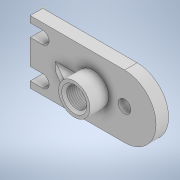
# Autodesk Inventor part: Деталь1
Saved by Autodesk Inventor 2020 (Build 240168000, 168)
## iProperties
Created: 2020-03-27
Part Number: Деталь1
Material: Типовые
Document SubType Name: Modeling
Designer: Trickster2038
Density: 1 g/cm^3
Appearance: По умолчанию
Mass: 46.5985 g
Surface Area: 144.743 cm^2
Volume: 46.5985 cm^3
Author: Trickster2038
Autodesk Inventor part; units mm, degrees
ref_plane "YZ Plane" through (0, 0, 0) normal (1, 0, 0) x (0, 1, 0)
sketch "Эскиз1" plane through (0, 0, 0) normal (0, 0, 1) x (1, 0, 0)
  line L0 (0, 0) -> (75, 0)
  line L1 (75, -50) -> (0, -50)
  line L2 (0, -50) -> (0, -45)
  arc A0 (75, -50) -> (75, 0) centre (75, -25) ccw
  line L3 (0, -25) -> (0, -15)
  line L4 (0, -15) -> (0, -35)
  line L5 (0, -35) -> (10, -35)
  line L6 (10, -45) -> (0, -45)
  line L7 (0, -15) -> (10, -15)
  line L8 (10, -5) -> (0, -5)
  arc A1 (10, -15) -> (10, -5) centre (10, -10) ccw
  arc A2 (10, -45) -> (10, -35) centre (10, -40) ccw
  line L9 (0, -5) -> (0, 0)
  line L10 (0, -35) -> (0, -15)
  circle A3 centre (50, -25) radius 12.5
  circle A4 centre (75, -25) radius 5
  line L11 (20, -25) -> (20, -21.5)
  line L12 (20, -21.5) -> (20, -28.5)
  line L13 (20, -28.5) -> (38, -28.5)
  line L14 (20, -21.5) -> (38, -21.5)
  constraints: 30 end point, 8 point on circle, 7 perpendicular, 5 centre point, 2 horizontal, 2 parallel, 1 coincident, 1 point on line, 1 vertical
sketch "Эскиз2" plane through (0, 0, 0) normal (0, 1, 0) x (-1, 0, 0)
  point P0 (0, 0)
sketch "Эскиз3" plane through (0, 0, 0) normal (0, 1, 0) x (-1, 0, 0)
  line L0 (0, 0) -> (0, 10)
  line L1 (0, 10) -> (-20, 10)
  line L2 (-20, 10) -> (-37.5, 10)
  line L3 (-37.5, 10) -> (-37.5, 20)
  line L4 (-37.5, 20) -> (-20, 10)
  line L5 (-44.031, 23.732) -> (-37.5, 20)
  line L6 (-44.031, 23.732) -> (-44.031, 33.732)
  line L7 (-44.031, 33.732) -> (-20, 33.732)
  line L8 (-20, 33.732) -> (-20, 10)
  dimension "d24" = 10
  dimension "d25" = 20
  dimension "d26" = 17.5
  dimension "d27" = 10
  dimension "d28" = 10
  constraints: 18 end point, 3 perpendicular, 2 point on line, 2 vertical, 1 collinear, 1 parallel
  measures "d24" distance of L0.start L0.end
  measures "d25" distance of L0.end L1.end
  measures "d26" distance of L1.end L2.end
  measures "d27" distance of L2.end L3.end
  measures "d28" distance of L5.start L6.end
sketch "Эскиз4" plane through (0, 0, 0) normal (0, 1, 0) x (-1, 0, 0)
  point P0 (0, 0)
ref_plane "РабПлоскость1" through (0, 0, 0) normal (0, 0, 1) x (1, 0, 0)
sketch "Эскиз5" plane through (0, 0, 0) normal (0, 0, 1) x (1, 0, 0)
  circle A0 centre (50, -25) radius 12.5
  point P0 (0, 0)
  constraints: 1 centre point
ref_plane "РабПлоскость2" through (0, 0, 0) normal (0, 0, 1) x (1, 0, 0)
sketch "Эскиз6" plane through (0, 0, 0) normal (0, 0, 1) x (1, 0, 0)
  line L0 (20, -21.5) -> (20, -28.5)
  line L1 (20, -28.5) -> (39.2288, -28.5)
  line L2 (39.2288, -28.5) -> (39.2288, -21.5)
  line L3 (39.2288, -21.5) -> (20, -21.5)
  point P0 (0, 0)
  constraints: 8 end point, 3 perpendicular, 1 vertical
extrude "Выдавливание1" add sketch "Эскиз1" along normal blind 10
extrude "Выдавливание2" add sketch "Эскиз6" along normal blind 25
extrude "Выдавливание3" cut sketch "Эскиз3" against normal blind 35 contours L4 L5 L6 L7 L8
ref_plane "РабПлоскость3" through (0, 0, 0) normal (0, 0, 1) x (1, 0, 0)
sketch "Эскиз7" plane through (0, 0, 0) normal (0, 0, 1) x (1, 0, 0)
  circle A0 centre (50, -25) radius 12.5
  point P0 (0, 0)
  constraints: 1 centre point
extrude "Выдавливание4" cut sketch "Эскиз7" along normal blind 25
extrude "Выдавливание5" add sketch "Эскиз5" along normal blind 25
ref_plane "РабПлоскость4" through (0, 0, 40) normal (0, 0, 1) x (1, 0, 0)
sketch "Эскиз8" plane through (0, 0, 40) normal (0, 0, 1) x (1, 0, 0)
  circle A0 centre (50, -25) radius 8
  point P0 (0, 0)
  constraints: 1 centre point
extrude "Выдавливание6" cut sketch "Эскиз8" against normal blind 70
thread "Резьба1" size "M16x1.5" class "6H" standard "ANSI Metric M Profile" full length
chamfer "Фаска1" distance 2 angle 45 1 edges at (42, -25, 25)
